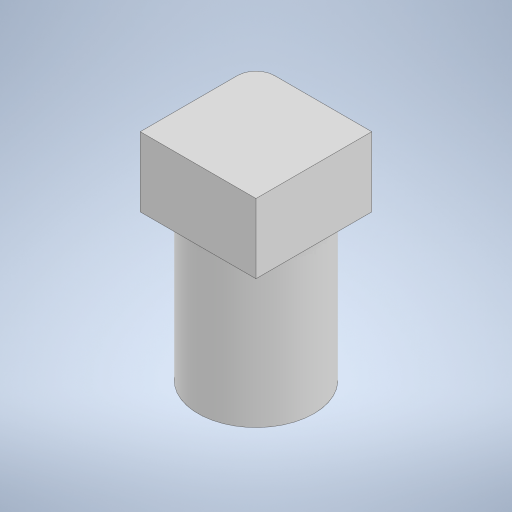
# Autodesk Inventor part: rotator_flat
Saved by Autodesk Inventor 2023.1 (Build 271208000, 208)
## iProperties
Created: 2022-10-07
Part Number: rotator_flat
Material: Generic
Document SubType Name: Modeling
Designer: swang
Density: 1 g/cm^3
Appearance: Default
Author: swang
## iProperties of the stored document rotator_round_3DPrint.ipt
Created: 2022-10-07
Part Number: rotator_round_3DPrint
Material: Generic
Document SubType Name: Modeling
Designer: swang
Density: 1 g/cm^3
Appearance: Default
Author: swang
Autodesk Inventor part; units mm, degrees
ref_plane "YZ Plane" through (0, 0, 0) normal (1, 0, 0) x (0, 1, 0)
ref_plane "XZ Plane" through (0, 0, 0) normal (0, 1, 0) x (-1, 0, 0)
ref_plane "XY Plane" through (0, 0, 0) normal (0, 0, 1) x (1, 0, 0)
sketch "Sketch1" plane through (0, 0, 0) normal (0, 1, 0) x (-1, 0, 0)
  circle A0 centre (0, 0) radius 25
  dimension "d0" = 50
  constraints: 1 centre point, 1 coincident
  measures "d0" diameter of A0
extrude "Extrusion1" add sketch "Sketch1" along normal blind 80
sketch "Sketch6" plane through (0, 80, 0) normal (0, 1, 0) x (1, 0, 0)
  line L0 (-8, 8) -> (42, 8)
  line L1 (42, 8) -> (42, -42)
  line L2 (42, -42) -> (-8, -42)
  line L3 (-8, -42) -> (-8, 8)
  point P0 (0, 0)
  dimension "d15" = 50
  dimension "d16" = 50
  dimension "d17" = 8
  dimension "d18" = 8
  constraints: 8 end point, 2 parallel, 1 horizontal, 1 perpendicular
  measures "d15" distance of L2.end L0.start
  measures "d16" distance of L1.end L2.end
  measures "d17" distance from line of point (0, 0) L3
  measures "d18" distance from line of L0 point (0, 0)
extrude "Extrusion4" add sketch "Sketch6" along normal blind 30
fillet "Fillet1" radius 8 1 edges at (-8, 95, -8)
body "Solid1"
